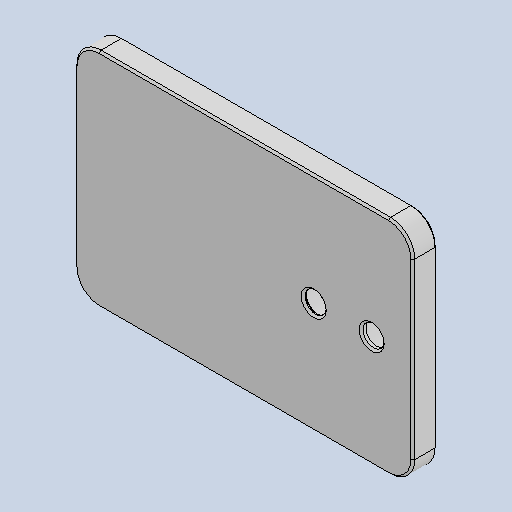
# Autodesk Inventor part: Takumar-foot-flat
Saved by Autodesk Inventor 2026 (Build 300175050, 175E)
## iProperties
Created: 2025-11-07
Part Number: Takumar-foot-flat
Material: Generic
Document SubType Name: Modeling
Designer: kuzmin
Density: 1 g/cm^3
Appearance: Default
Author: kuzmin
Autodesk Inventor part; units mm, degrees
ref_plane "YZ Plane" through (0, 0, 0) normal (1, 0, 0) x (0, 1, 0)
ref_plane "XZ Plane" through (0, 0, 0) normal (0, 1, 0) x (-1, 0, 0)
ref_plane "XY Plane" through (0, 0, 0) normal (0, 0, 1) x (1, 0, 0)
sketch "Sketch1" plane through (0, 0, 0) normal (0, 0, 1) x (1, 0, 0)
  line L0 (-35, 23) -> (35, 23)
  line L1 (35, 23) -> (35, -23)
  line L2 (35, -23) -> (-35, -23)
  line L3 (-35, -23) -> (-35, 23)
  point P0 (0, 0)
  point P1 (0, 23)
  point P2 (35, 0)
  dimension "d0" = 46
  dimension "d1" = 70
  constraints: 8 end point, 2 midpoint, 2 parallel, 1 horizontal, 1 horizontal alignment, 1 perpendicular, 1 vertical alignment
  measures "d0" distance of L0.end L1.end
  measures "d1" distance of L0.start L0.end
extrude "Extrusion1" add sketch "Sketch1" along normal blind 5
sketch "Sketch3" plane through (0, 0, 0) normal (0, 0, -1) x (-1, 0, 0)
  line L0 (-26.46, 0) -> (-14.46, 0) construction
  line L1 (-35, -23) -> (-35, 23) projected
  point P0 (0, 0)
  dimension "d7" = 12
  dimension "d8" = 8.54
  constraints: 2 coincident, 2 end point, 1 horizontal
  measures "d7" distance of L0.start L0.end
  measures "d8" distance from line of point (-26.46, 0) L1
hole "Hole1" at (14.46, 0, 0) at (26.46, 0, 0) direction (0, 0, 1) diameter 4.4 end through all counterbore diameter 8 counterbore depth 4
fillet "Fillet1" radius 5 4 edges at (35, -23, 2.5) (35, 23, 2.5) (-35, 23, 2.5) (-35, -23, 2.5)
chamfer "Chamfer2" distance 0.4 angle 45 23 edges at (0, -23, 5) (33.5355, -21.5355, 5) (35, 0, 5) (33.5355, 21.5355, 5) (0, 23, 5) (-33.5355, 21.5355, 5) (-35, 0, 5) (-33.5355, -21.5355, 5) (0, -23, 0) (33.5355, -21.5355, 0) (35, 0, 0) (33.5355, 21.5355, 0) (0, 23, 0) (-33.5355, 21.5355, 0) (-35, 0, 0) (-33.5355, -21.5355, 0) (14.46, -4, 0) (26.46, -4, 0) (26.46, -2.2, 5) (14.46, -2.2, 5) (14.46, -2.2, 4) (14.46, -4, 4) (26.46, -4, 4)
equation "\"d2\" = thickness"
equation "\"thickness\" = 5"
body "Solid1"
